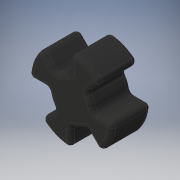
# Autodesk Inventor part: crabot
Saved by Autodesk Inventor 2018 (Build 220112000, 112)
## iProperties
Created: 2020-03-23
Part Number: crabot
Material: Generic
Document SubType Name: Modeling
Designer: emile
Density: 1 g/cm^3
Appearance: Rubber - Black
Author: emile
Autodesk Inventor part; units mm, degrees
ref_plane "YZ Plane" through (0, 0, 0) normal (1, 0, 0) x (0, 1, 0)
ref_plane "XZ Plane" through (0, 0, 0) normal (0, 1, 0) x (-1, 0, 0)
ref_plane "XY Plane" through (0, 0, 0) normal (0, 0, 1) x (1, 0, 0)
sketch "Sketch1" plane through (0, 0, 0) normal (0, 0, 1) x (1, 0, 0)
  circle A0 centre (0, 0) radius 7.9375
  circle A1 centre (0, 0) radius 4.1275
  line L0 (0, 7.9375) -> (0, 4.1275)
  arc A2 (2.9186, 2.9186) -> (0, 4.1275) centre (0, 0) ccw
  line L1 (2.9186, 2.9186) -> (5.6127, 5.6127)
  line L2 (0, 4.1275) -> (0, 0) construction
  line L3 (0, 0) -> (2.9186, 2.9186) construction
  dimension "d13" = 8.255
  dimension "d0" = 15.875
  dimension "d2" = 45
  constraints: 8 end point, 4 point on circle, 3 coincident, 2 centre point, 2 collinear, 1 vertical, 1 vertical alignment, 2 other
  measures "d0" diameter of A0
  measures "d2" angle of L1 L0
extrude "Extrusion3" add sketch "Sketch1" along normal blind 7.4581 contours L1 A1 L0 A0 | A1 picked at (4.3137, 5.0437)
fillet "Fillet3" radius 0.7937 4 edges at (0, 7.9375, 3.729) (5.6127, 5.6127, 3.729) (2.9186, 2.9186, 3.729) (0, 4.1275, 3.729)
pattern_circular "Circular Pattern2" count 4 over 360 about axis through (0, 0, 0) along (0, 0, 1) of "Fillet3", "Extrusion3"
fillet "Fillet4" radius 0.7937 64 edges at (4.2272, 4.2272, 7.4581) (3.2044, 2.9372, 7.4581) (3.8133, 1.5795, 7.4581) (4.3428, 0.1889, 7.4581) (5.9782, 0, 7.4581) (7.6911, -0.2646, 7.4581) (7.3333, -3.0375, 7.4581) (5.6255, -5.2514, 7.4581) (4.2272, -4.2272, 7.4581) (2.9372, -3.2044, 7.4581) (1.5795, -3.8133, 7.4581) (0.1889, -4.3428, 7.4581) (0, -5.9782, 7.4581) (-0.2646, -7.6911, 7.4581) (-3.0375, -7.3333, 7.4581) (-5.2514, -5.6255, 7.4581) (-4.2272, -4.2272, 7.4581) (-3.2044, -2.9372, 7.4581) (-3.8133, -1.5795, 7.4581) (-4.3428, -0.1889, 7.4581) (-5.9782, 0, 7.4581) (-7.6911, 0.2646, 7.4581) (-7.3333, 3.0375, 7.4581) (-5.6255, 5.2514, 7.4581) (-4.2272, 4.2272, 7.4581) (-2.9372, 3.2044, 7.4581) (-1.5795, 3.8133, 7.4581) (-0.1889, 4.3428, 7.4581) (0, 5.9782, 7.4581) (0.2646, 7.6911, 7.4581) (3.0375, 7.3333, 7.4581) (5.2514, 5.6255, 7.4581) (3.0375, 7.3333, 0) (0.2646, 7.6911, 0) (0, 5.9782, 0) (-0.1889, 4.3428, 0) (-1.5795, 3.8133, 0) (-2.9372, 3.2044, 0) (-4.2272, 4.2272, 0) (-5.6255, 5.2514, 0) (-7.3333, 3.0375, 0) (-7.6911, 0.2646, 0) (-5.9782, 0, 0) (-4.3428, -0.1889, 0) (-3.8133, -1.5795, 0) (-3.2044, -2.9372, 0) (-4.2272, -4.2272, 0) (-5.2514, -5.6255, 0) (-3.0375, -7.3333, 0) (-0.2646, -7.6911, 0) (0, -5.9782, 0) (0.1889, -4.3428, 0) (1.5795, -3.8133, 0) (2.9372, -3.2044, 0) (4.2272, -4.2272, 0) (5.6255, -5.2514, 0) (7.3333, -3.0375, 0) (7.6911, -0.2646, 0) (5.9782, 0, 0) (4.3428, 0.1889, 0) (3.8133, 1.5795, 0) (3.2044, 2.9372, 0) (4.2272, 4.2272, 0) (5.2514, 5.6255, 0)
body "Solid2"
